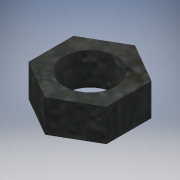
# Autodesk Inventor part: half-inch hex nut
Saved by Autodesk Inventor 2016 (Build 200138000, 138)
## iProperties
Created: 2016-01-17
Part Number: half-inch hex nut
Material: Steel
Document SubType Name: Modeling
Designer: gus
Density: 7.85 g/cm^3
Appearance: Plate
Mass: 4.93155 g
Surface Area: 6.83836 cm^2
Volume: 0.628223 cm^3
User Status: complete
Author: gus
Autodesk Inventor part; units mm, degrees
ref_plane "YZ Plane" through (0, 0, 0) normal (1, 0, 0) x (0, 1, 0)
ref_plane "XZ Plane" through (0, 0, 0) normal (0, 1, 0) x (-1, 0, 0)
ref_plane "XY Plane" through (0, 0, 0) normal (0, 0, 1) x (1, 0, 0)
sketch "Sketch1" plane through (0, 0, 0) normal (0, 1, 0) x (-1, 0, 0)
  line L0 (7.1437, -4.1244) -> (0, -8.2489)
  line L1 (0, -8.2489) -> (-7.1437, -4.1244)
  line L2 (-7.1437, -4.1244) -> (-7.1438, 4.1244)
  line L3 (-7.1438, 4.1244) -> (0, 8.2489)
  line L4 (0, 8.2489) -> (7.1438, 4.1244)
  line L5 (7.1438, 4.1244) -> (7.1437, -4.1244)
  circle A0 centre (0, 0) radius 4.7625
  dimension "d0" = 14.2875
  dimension "d1" = 9.525
  constraints: 12 end point, 2 coincident, 1 centre point, 1 vertical, 13 other
  measures "d0" distance between parallel lines of L2 L5
  measures "d1" diameter of A0
extrude "Extrusion1" add sketch "Sketch1" along normal blind 5.9531
body "Solid1"
